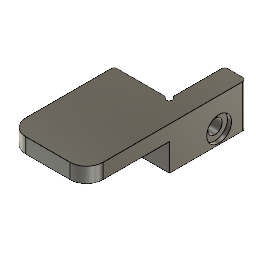
support_right (Autodesk Fusion 360 design; units mm, degrees)
Autodesk Fusion 360 part; units mm, degrees
note: some values were not read from the file. Chosen so that the rebuilt part matches the saved one: which face or edge a step refers to. Set by a fixed rule: which sketch regions a step uses.
sketch "Sketch1" plane through (0, 0, 0) normal (0, 0, 1) x (1, 0, 0) in component "support"
  circle A0 centre (0, 0) radius 4
  line L0 (-6.35, -6.35) -> (21.65, -6.35)
  line L1 (21.65, -6.35) -> (21.65, 51.65)
  line L2 (21.65, 51.65) -> (13.65, 51.65)
  line L3 (13.65, 51.65) -> (13.65, 31.65)
  line L4 (13.65, 31.65) -> (-6.35, 31.65)
  line L5 (-6.35, 31.65) -> (-6.35, -6.35)
  circle A1 centre (13.65, 31.65) radius 1
  line L6 (21.65, 23.65) -> (-6.35, 23.65)
  dimension "d1" = 8
  dimension "d2" = 2
  dimension "d3" = 20
  dimension "d4" = 20
  dimension "d5" = 8
  dimension "d6" = 21.65
  dimension "d7" = 31.65
  dimension "d15" = 8
  dimension "d31" = 58
  measures "d1" diameter of A0
  measures "d2" diameter of A1
  measures "d5" distance of A0.centre
  measures "d6" distance of A0.centre L1
  measures "d7" distance of A0.centre L4
  measures "d15" distance of L4 L6
  measures "d31" distance of A0.centre
extrude "Extrude1" add sketch "Sketch1" along normal blind 1.5 contours A0 | L0 L1 L5 L6 | L1 L2 L3 L4 L5 A1 L6 in component "support"
extrude "Extrude2" add sketch "Sketch1" against normal blind 4 contours L0 L1 L5 L6 | L1 L2 L3 L4 L5 A1 L6 in component "support"
extrude "Extrude3" add sketch "Sketch1" against normal blind 10 from surface at -4 contours L1 L2 L3 L4 L5 A1 L6 in component "support"
sketch "side hole" plane through (21.65, 0, 0) normal (1, 0, 0) x (0, 1, 0) in component "support"
  line L0 (31.65, -14) -> (31.65, 1.5)
  line L1 (31.65, 1.5) -> (31.65, -14)
  line L2 (51.65, -9) -> (31.65, -9) construction
  line L3 (23.65, -4) -> (-6.35, -4)
  line L4 (-6.35, -4) -> (23.65, -4)
  line L5 (4, -4) -> (-4, -4)
  line L6 (23.65, -4) -> (31.65, -4) construction
  line L7 (31.65, -4) -> (31.65, -14) construction
  dimension "d12" = 20
hole "Hole1" at (21.65, 41.65, -9) direction (-1, 0, 0) diameter 5.2 depth 8 tip angle 180 counterbore diameter 9 counterbore depth 1.5 in component "support"
sketch "Sketch6" plane through (0, 23.65, 0) normal (0, -1, 0) x (1, 0, 0) in component "support"
  line L0 (13.65, -11.6) -> (13.65, -6.4)
  line L1 (13.65, -14) -> (13.65, 1.5)
  line L2 (13.65, 1.5) -> (13.65, -14)
  line L3 (-6.35, -4) -> (21.65, -4)
  line L4 (21.65, -4) -> (-6.35, -4)
  line L5 (4, -4) -> (-4, -4)
  line L6 (13.65, -4) -> (13.65, -14) construction
  line L7 (13.65, -9) -> (-6.35, -9) construction
  dimension "d25" = 20
hole "Hole2" at (3.65, 23.65, -9) direction (0, 1, 0) diameter 5.2 depth 8 tip angle 180 counterbore diameter 9 counterbore depth 1.5 in component "support"
fillet "Fillet1" radius 6 2 edges at (-6.35, -6.35, -1.25) (21.65, -6.35, -1.25) in component "support"
fillet "Fillet2" radius 1.5 1 edges at (21.65, 51.65, -6.25) in component "support"
fillet "Fillet3" radius 1 2 edges at (13.65, 51.65, -6.25) (-6.35, 31.65, -6.25) in component "support"
fillet "Fillet4" radius 1 2 edges at (13.65, 32.65, -6.25) (12.65, 31.65, -6.25) in component "support"
component "support" placed x (1, 0, 0) y (0, 1, 0) z (0, 0, 1) at (0, 0, 0)
